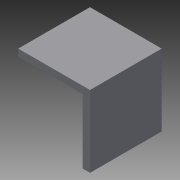
# Autodesk Inventor part: dociskacz
Saved by Autodesk Inventor 2015 (Build 190159000, 159)
## iProperties
Created: 2015-05-04
Part Number: dociskacz
Material: Ogólny
Document SubType Name: Modeling
Designer: Kuba
Density: 1 g/cm^3
Appearance: Domyślna
Author: Kuba
Autodesk Inventor part; units mm, degrees
ref_plane "YZ Plane" through (0, 0, 0) normal (1, 0, 0) x (0, 1, 0)
ref_plane "XZ Plane" through (0, 0, 0) normal (0, 1, 0) x (-1, 0, 0)
ref_plane "XY Plane" through (0, 0, 0) normal (0, 0, 1) x (1, 0, 0)
sketch "Szkic1" plane through (0, 0, 0) normal (0, 1, 0) x (-1, 0, 0)
  line L0 (0, 0) -> (20, 0)
  line L1 (0, -20) -> (0, 0)
  line L2 (20, 0) -> (20, -2)
  line L3 (20, -2) -> (2, -2)
  line L4 (2, -2) -> (2, -20)
  line L5 (2, -20) -> (0, -20)
  dimension "d2" = 2
  dimension "d3" = 18
  dimension "d4" = 20
  dimension "d5" = 18
  dimension "d6" = 2
  constraints: 12 end point, 3 perpendicular, 2 horizontal
  measures "d2" distance of L0.end L2.end
  measures "d3" distance of L2.end L3.end
  measures "d4" distance of L1.start L0.start
  measures "d5" distance of L3.end L4.end
  measures "d6" distance of L4.end L1.start
extrude "Wyciągnięcie proste1" add sketch "Szkic1" along normal blind 20
